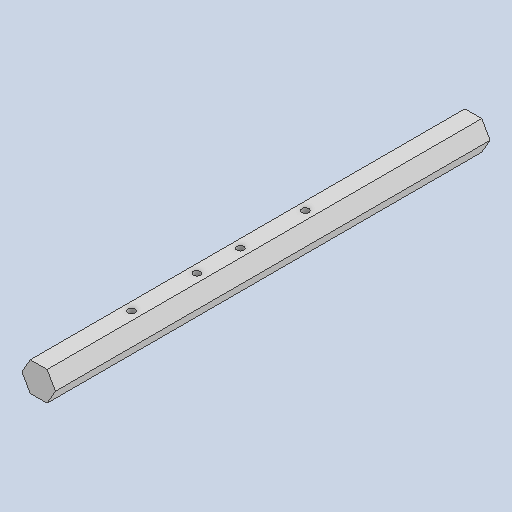
# Autodesk Inventor part: Eje2
Saved by Autodesk Inventor 2022 (Build 260153000, 153)
## iProperties
Created: 2022-02-21
Part Number: Eje2
Material: Generic
Document SubType Name: Modeling
Designer: katha
Density: 1 g/cm^3
Appearance: Default
Author: katha
Autodesk Inventor part; units mm, degrees
ref_plane "YZ Plane" through (0, 0, 0) normal (1, 0, 0) x (0, 1, 0)
ref_plane "XZ Plane" through (0, 0, 0) normal (0, 1, 0) x (-1, 0, 0)
ref_plane "XY Plane" through (0, 0, 0) normal (0, 0, 1) x (1, 0, 0)
sketch "Sketch5" plane through (0, 0, 0) normal (0, 0, 1) x (1, 0, 0)
  line L0 (0, 0) -> (3.1, 0) construction
  circle A0 centre (0, 0) radius 3.1 construction
  line L1 (0, 0) -> (1.55, 2.6847) construction
  line L2 (0, 0) -> (-1.55, 2.6847) construction
  line L3 (0, 0) -> (-3.1, 0) construction
  line L4 (0, 0) -> (-1.55, -2.6847) construction
  line L5 (0, 0) -> (1.55, -2.6847) construction
  line L6 (-1.55, 2.6847) -> (1.55, 2.6847)
  line L7 (1.55, 2.6847) -> (3.1, 0)
  line L8 (3.1, 0) -> (1.55, -2.6847)
  line L9 (1.55, -2.6847) -> (-1.55, -2.6847)
  line L10 (-1.55, -2.6847) -> (-3.1, 0)
  line L11 (-3.1, 0) -> (-1.55, 2.6847)
  dimension "d9" = 3.1
  dimension "d12" = 360
  constraints: 24 end point, 3 point on circle, 2 horizontal, 2 parallel, 1 centre point, 1 coincident, 1 point on line, 19 other
  measures "d9" distance of L0.start L0.end
extrude "Extrusion5" add sketch "Sketch5" along normal blind 80
sketch "Sketch6" plane through (-1.55, 2.6847, 0) normal (0, 1, 0) x (1, 0, 0)
  line L0 (3.1, -80) -> (0, -80) construction
  line L1 (3.1, 0) -> (0, 0) construction
  line L2 (0, -80) -> (3.1, -80) construction
  line L3 (1.55, -80) -> (1.55, 0) construction
  line L4 (3.1, 0) -> (3.1, -80) projected
  circle A0 centre (1.55, -30.9) radius 0.65
  circle A1 centre (1.55, -42.9) radius 0.65
  circle A2 centre (1.55, -50.9) radius 0.65
  circle A3 centre (1.55, -62.9) radius 0.65
  dimension "d16" = 1.3
  dimension "d17" = 49.1
  dimension "d18" = 37.1
  dimension "d19" = 29.1
  dimension "d20" = 17.1
  constraints: 4 centre point, 4 point on line, 3 equal radius, 2 end point, 1 midpoint, 1 parallel
  measures "d16" diameter of A0
  measures "d17" distance from line of A0.centre L0
  measures "d18" distance from line of A1.centre L0
  measures "d19" distance from line of A2.centre L0
  measures "d20" distance from line of A3.centre L0
extrude "Extrusion6" cut sketch "Sketch6" against normal blind 6
body "Solid2"
